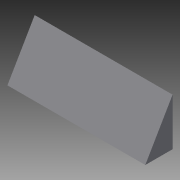
# Autodesk Inventor part: Pickup ramp Idea
Saved by Autodesk Inventor 2014 SP1 (Build 180222100, 222)
## iProperties
Created: 2014-01-18
Part Number: Pickup ramp Idea
Material: Generic
Document SubType Name: Modeling
Designer: Paul
Density: 1 g/cm^3
Appearance: Default
Author: Paul
Autodesk Inventor part; units mm, degrees
ref_plane "YZ Plane" through (0, 0, 0) normal (1, 0, 0) x (0, 1, 0)
ref_plane "XZ Plane" through (0, 0, 0) normal (0, 1, 0) x (-1, 0, 0)
ref_plane "XY Plane" through (0, 0, 0) normal (0, 0, 1) x (1, 0, 0)
sketch "Sketch1" plane through (0, 0, 0) normal (1, 0, 0) x (0, 1, 0)
  line L0 (0, 0) -> (147.955, 0)
  line L1 (147.955, 0) -> (0, 85.4202)
  line L2 (0, 85.4202) -> (0, 0)
  dimension "d0" = 85.4202
  dimension "d1" = 147.955
  constraints: 6 end point, 1 horizontal, 1 perpendicular
  measures "d0" distance of L1.end L0.start
  measures "d1" distance of L0.start L0.end
extrude "Extrusion1" add sketch "Sketch1" along normal blind 431.8
body "Solid1"
